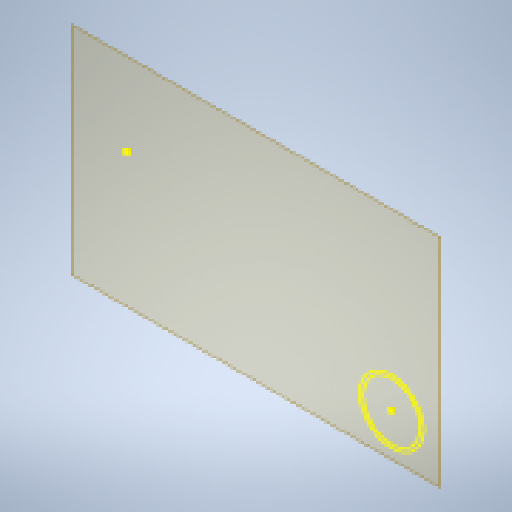
# Autodesk Inventor part: WashChamberConduit
Saved by Autodesk Inventor 2024 (Build 280153000, 153)
## iProperties
Created: 2024-09-07
Part Number: WashChamberConduit
Material: Generic
Document SubType Name: Modeling
Designer: Tommy Rohmann
Density: 1 g/cm^3
Appearance: Default
Author: Tommy Rohmann
Autodesk Inventor part; units mm, degrees
ref_plane "YZ Plane" through (0, 0, 0) normal (1, 0, 0) x (0, 1, 0)
ref_plane "XZ Plane" through (0, 0, 0) normal (0, 1, 0) x (-1, 0, 0)
ref_plane "XY Plane" through (0, 0, 0) normal (0, 0, 1) x (1, 0, 0)
ref_plane "Work Plane1" through (68.3233, -161.4118, -30.3466) normal (0, 1, 0) x (1, 0, 0)
sketch "Sketch1" plane through (68.3233, -161.4118, -30.3466) normal (0, 1, 0) x (1, 0, 0)
  circle A0 centre (403.7379, -91.8941) radius 62.1665 construction
  line L0 (403.7379, -91.8941) -> (479.9379, -91.8941) construction
  line L1 (454.5379, -91.8941) -> (454.5379, -88.7191)
  line L2 (454.5379, -91.8941) -> (454.5379, 25.7495) construction
  line L3 (460.8879, 419.2809) -> (460.8879, 25.7495) construction
  line L4 (465.9044, -162.549) -> (465.9044, 25.7495) construction
  line L5 (479.9379, -162.549) -> (479.9379, 25.7495) construction
  line L6 (454.5379, -88.7191) -> (465.9044, -88.7191)
  line L7 (465.9044, -88.7191) -> (465.9044, -82.3691)
  line L8 (461.2054, -91.8941) -> (461.2054, 25.7495) construction
  line L9 (465.9044, -82.3691) -> (461.2054, -82.3691)
  line L10 (461.2054, -82.3691) -> (461.2054, -77.3526)
  line L11 (461.2054, -77.3526) -> (465.9044, -77.3526)
  line L12 (465.9044, -72.3361) -> (461.2054, -72.3361)
  line L13 (465.9044, -67.3196) -> (461.2054, -67.3196)
  line L14 (465.9044, -77.3526) -> (465.9044, -72.3361)
  line L15 (461.2054, -72.3361) -> (461.2054, -67.3196)
  line L16 (465.9044, -62.3031) -> (461.2054, -62.3031)
  line L17 (465.9044, -67.3196) -> (465.9044, -62.3031)
  line L18 (461.2054, -62.3031) -> (461.2054, -57.2866)
  line L19 (461.2054, -57.2866) -> (479.9379, -57.2866)
  line L20 (479.9379, -116.9766) -> (403.7379, -116.9766) construction
  line L21 (454.5379, -91.8941) -> (463.5549, -116.9766)
  line L22 (463.5549, -116.9766) -> (479.9379, -116.9766)
  line L23 (479.9379, -116.9766) -> (479.9379, -57.2866)
  line L24 (403.7379, -91.8941) -> (403.7379, 17.9547)
  line L25 (467.2379, 419.2809) -> (340.2379, 419.2809) projected
  line L26 (352.9379, -88.7191) -> (454.5379, -88.7191) projected
  point P0 (-68.3233, -30.3466)
  dimension "d11" = 3.175
  dimension "d13" = 0.3175
  dimension "d23" = 25.0825
  dimension "d25" = 76.2
  dimension "d26" = 5.0165
  dimension "d27" = 9.017
  constraints: 48 end point, 16 point on line, 9 perpendicular, 7 vertical, 4 collinear, 1 centre point, 1 horizontal, 1 parallel, 1 tangent, 8 other
  measures "d11" distance of L1.start L1.end
  measures "d13" distance between parallel lines of L3 L8
  measures "d25" distance from line of A0.centre L5
  measures "d26" distance between parallel lines of L3 L4
  measures "d27" horizontal distance of L21.end L1.start
revolve "Revolution1" add sketch "Sketch1" angle 360 about axis through (472.0613, -161.4118, 61.5475) along (0, 0, -1)
ref_plane "Work Plane5" through (925.2638, -75.6868, 84.6043) normal (0, 1, 0) x (0.2885633, 0, 0.9574608)
sketch "Sketch3" plane through (925.2638, -75.6868, 84.6043) normal (0, 1, 0) x (0.2885633, 0, 0.9574608)
  line L0 (15.1158, -271.5524) -> (15.1158, -268.3774)
  line L1 (15.1158, -268.3774) -> (26.4823, -268.3774)
  line L2 (26.4823, -268.3774) -> (26.4823, -262.0274)
  line L3 (26.4823, -262.0274) -> (21.7833, -262.0274)
  line L4 (21.7833, -262.0274) -> (21.7833, -257.0109)
  line L5 (21.7833, -257.0109) -> (26.4823, -257.0109)
  line L6 (26.4823, -251.9944) -> (21.7833, -251.9944)
  line L7 (26.4823, -246.9779) -> (21.7833, -246.9779)
  line L8 (26.4823, -257.0109) -> (26.4823, -251.9944)
  line L9 (21.7833, -251.9944) -> (21.7833, -246.9779)
  line L10 (26.4823, -241.9614) -> (21.7833, -241.9614)
  line L11 (26.4823, -246.9779) -> (26.4823, -241.9614)
  line L12 (21.7833, -241.9614) -> (21.7833, -236.9449)
  line L13 (21.7833, -236.9449) -> (40.5158, -236.9449)
  line L14 (15.1158, -271.5524) -> (24.1328, -296.6349)
  line L15 (24.1328, -296.6349) -> (40.5158, -296.6349)
  line L16 (40.5158, -296.6349) -> (40.5158, -236.9449)
  point P0 (-348.0025, -861.4902)
  point P1 (15.1158, -268.3774)
  dimension "d29" = 3.175
  dimension "d30" = 9.017
  constraints: 34 end point
  measures "d29" distance of L0.start L1.start
  measures "d30" horizontal distance of L14.end L0.start
equation "\"d23\" = 5 * d26"
body "Solid1"
